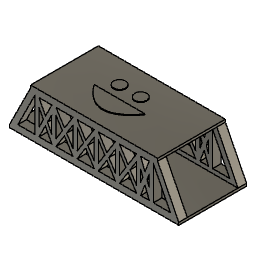
jason (Autodesk Fusion 360 design; units mm, degrees)
Autodesk Fusion 360 part; units mm, degrees
sketch "Sketch1" plane through (0, 0, 0) normal (0, 0, 1) x (1, 0, 0)
  line L0 (-100, 0) -> (-75, 50)
  line L1 (-75, 50) -> (75, 50)
  line L2 (75, 50) -> (100, 0)
  line L3 (100, 0) -> (-100, 0)
  line L4 (-70, 45) -> (-90, 5)
  line L5 (-90, 5) -> (90, 5)
  line L6 (90, 5) -> (70, 45)
  line L7 (70, 45) -> (-70, 45)
  line L8 (-70, 45) -> (-70, 5)
  line L9 (-50, 45) -> (-70, 5)
  line L10 (-50, 45) -> (-50, 5)
  line L11 (-50, 45) -> (-50, 5)
  line L12 (-50, 5) -> (-30, 45)
  line L13 (-30, 45) -> (-30, 5)
  line L14 (-10, 45) -> (-30, 5)
  line L15 (-10, 45) -> (-10, 5)
  line L16 (10, 45) -> (-10, 5)
  line L17 (10, 45) -> (10, 5)
  line L18 (10, 5) -> (30, 45)
  line L19 (30, 5) -> (30, 45)
  line L20 (30, 5) -> (50, 45)
  line L21 (50, 5) -> (50, 45)
  line L22 (70, 45) -> (50, 5)
  line L23 (70, 45) -> (70, 5)
  line L24 (-50, 5) -> (-60, 25)
  line L25 (-40, 25) -> (-30, 5)
  line L26 (-20, 25) -> (-10, 5)
  line L27 (0, 25) -> (10, 5)
  line L28 (20, 25) -> (30, 5)
  line L29 (40, 25) -> (50, 5)
  line L30 (60, 25) -> (70, 5)
  line L31 (80, 25) -> (70, 5)
  line L32 (-70, 6.8562) -> (-80, 25)
  line L33 (-70, 45) -> (-60, 25)
  line L34 (-50, 45) -> (-40, 25)
  line L35 (-30, 45) -> (-20, 25)
  line L36 (-10, 45) -> (0, 25)
  line L37 (10, 45) -> (20, 25)
  line L38 (30, 45) -> (40, 25)
  line L39 (50, 45) -> (60, 25)
  line L40 (-80, 25) -> (80, 25)
  constraint horizontal L1
  constraint parallel L1 L3
  constraint parallel L0 L4
  constraint parallel L3 L5
  constraint parallel L1 L7
  constraint coincident L5 L8.end
  constraint perpendicular L5 L8
  constraint coincident L7 L9.start
  constraint coincident L5 L10.end
  constraint perpendicular L5 L10
  constraint perpendicular L5 L11
  constraint coincident L7 L12.end
  constraint parallel L9 L12
  constraint coincident L5 L13.end
  constraint perpendicular L5 L13
  constraint coincident L7 L14.start
  constraint parallel L12 L14
  constraint coincident L5 L15.end
  constraint perpendicular L5 L15
  constraint coincident L7 L16.start
  constraint parallel L14 L16
  constraint coincident L5 L17.end
  constraint perpendicular L7 L17
  constraint coincident L7 L18.end
  constraint parallel L16 L18
  constraint coincident L5 L19.start
  constraint perpendicular L7 L19
  constraint coincident L7 L20.end
  constraint coincident L5 L21.start
  constraint perpendicular L7 L21
  constraint parallel L20 L22
  constraint coincident L5 L23.end
  constraint perpendicular L5 L23
  constraint midpoint L9 L24.end
  constraint midpoint L12 L25.start
  constraint midpoint L14 L26.start
  constraint midpoint L16 L27.start
  constraint midpoint L18 L28.start
  constraint midpoint L20 L29.start
  constraint parallel L28 L29
  constraint midpoint L22 L30.start
  constraint midpoint L6 L31.start
  constraint coincident L8 L32.start
  constraint midpoint L4 L32.end
extrude "Extrude1" add sketch "Sketch1" along normal blind 10 makes body 1
move_face "MoveFace1" to x (0.8, 0.4, -0.447214) y (0.4, 0.2, 0.894427) z (0.447214, -0.894427, 0) at (2.6343, -5.2686, 5.8905) 1 faces at (83.3333, 33.3333, 3.3333) on bodies 1
move_body "Move1" bodies 1 to x (1, 0, 0) y (0, 0, 1) z (0, -1, 0) at (0, 15, 5)
move_body "Move2" bodies 1 to x (1, 0, 0) y (0, 1, 0) z (0, 0, 1) at (0, -10, -5)
sketch "Sketch2" plane through (0, 0, 0) normal (0, 1, 0) x (1, 0, 0)
  line L0 (-70, -45) -> (-70, -5)
  line L1 (-70, -5) -> (-65, -5)
  line L2 (-65, -5) -> (-65, -45)
  line L3 (-65, -45) -> (-70, -45)
  line L4 (-65, -45) -> (-45, -5)
  line L5 (-45, -5) -> (-50, -5)
  line L6 (-50, -5) -> (-70, -45)
  line L7 (-45, -5) -> (-45, -45)
  line L8 (-45, -45) -> (-50, -45)
  line L9 (-50, -45) -> (-50, -5)
  line L10 (-70, -5) -> (-50, -45)
  line L11 (-45, -45) -> (-51.984, -45)
  line L12 (-65, -5) -> (-45, -45)
  line L13 (-70, -5) -> (-65, -5)
  line L14 (-45, -45) -> (-50, -45)
  line L15 (-50, -45) -> (-25, -5)
  line L16 (-25, -5) -> (-20, -5)
  line L17 (-20, -5) -> (-45, -45)
  line L18 (-25, -45) -> (-25, -5)
  line L19 (-20, -5) -> (-20, -45)
  line L20 (-20, -45) -> (-25, -45)
  line L21 (-25, -45) -> (-50, -5)
  line L22 (-20, -45) -> (-45, -5)
  line L23 (-25, -45) -> (0, -5)
  line L24 (0, -5) -> (5, -5)
  line L25 (5, -5) -> (-20, -45)
  line L26 (5, -5) -> (5, -45)
  line L27 (5, -45) -> (-20, -5)
  line L28 (-25, -5) -> (0, -45)
  line L29 (0, -45) -> (5, -45)
  line L30 (0, -5) -> (0, -45)
  line L31 (0, -45) -> (25, -5)
  line L32 (25, -5) -> (30, -5)
  line L33 (30, -5) -> (5, -45)
  line L34 (30, -5) -> (30, -45)
  line L35 (30, -45) -> (25, -45)
  line L36 (25, -45) -> (25, -5)
  line L37 (0, -5) -> (25, -45)
  line L38 (5, -5) -> (30, -45)
  line L39 (25, -45) -> (50, -5)
  line L40 (50, -5) -> (55, -5)
  line L41 (55, -5) -> (30, -45)
  line L42 (50, -45) -> (50, -5)
  line L43 (55, -5) -> (55, -45)
  line L44 (55, -45) -> (50, -45)
  line L45 (55, -45) -> (30, -5)
  line L46 (50, -45) -> (25, -5)
  line L47 (55, -5) -> (70, -45)
  line L48 (70, -45) -> (70, -5)
  line L49 (70, -5) -> (65, -5)
  line L50 (65, -5) -> (65, -45)
  line L51 (65, -45) -> (70, -45)
  line L52 (55, -45) -> (70, -5)
  line L53 (50, -45) -> (65, -5)
  line L54 (65, -45) -> (50, -5)
  constraint vertical L0
  constraint perpendicular L0 L1
  constraint perpendicular L1 L2
  constraint perpendicular L0 L3
  constraint perpendicular L0 L5
  constraint parallel L4 L6
  constraint perpendicular L5 L7
  constraint perpendicular L7 L8
  constraint perpendicular L5 L9
  constraint perpendicular L9 L11
  constraint perpendicular L9 L16
  constraint parallel L15 L17
  constraint perpendicular L16 L18
  constraint perpendicular L16 L19
  constraint perpendicular L18 L20
  constraint perpendicular L19 L24
  constraint parallel L23 L25
  constraint perpendicular L24 L26
  constraint parallel L27 L28
  constraint perpendicular L26 L29
  constraint perpendicular L30 L32
  constraint parallel L31 L33
  constraint perpendicular L32 L34
  constraint perpendicular L34 L35
  constraint perpendicular L32 L36
  constraint perpendicular L34 L40
  constraint parallel L39 L41
  constraint perpendicular L40 L42
  constraint perpendicular L40 L43
  constraint perpendicular L42 L44
  constraint parallel L43 L48
  constraint perpendicular L49 L50
  constraint perpendicular L43 L51
  constraint parallel L52 L53
extrude "Extrude2" add sketch "Sketch2" against normal blind 5 contours L2 L3 L6 | L0 L2 L6 L10 | L1 L2 L10 L13 | L2 L4 L6 L10 | L2 L6 L10 L12 | L4 L6 L10 L12 | L4 L9 L10 L12 | L4 L6 L9 L12 | L8 L11 L12 L14 L15 | L9 L12 L15 | L4 L9 L21 | L4 L5 L21 | L4 L7 L9 L12 L15 L21 | L7 L12 L15 | L7 L15 L17 L21 | L4 L7 L21 | L7 L15 L21 L22 | L15 L17 L21 L22 | L17 L18 L21 L22 | L15 L17 L18 L22 | L20 L22 L23 | L18 L22 L23 | L17 L18 L28 | L16 L17 L28 | L17 L18 L19 L22 L23 L28 | L19 L22 L23 | L19 L23 L25 L28 | L17 L19 L28 | L19 L23 L27 L28 | L23 L25 L27 L28 | L25 L27 L28 L30 | L23 L25 L27 L30 | L27 L29 L31 | L27 L30 L31 | L25 L30 L37 | L24 L25 L37 | L25 L26 L27 L30 L31 L37 | L26 L27 L31 | L26 L31 L33 L37 | L25 L26 L37 | L26 L31 L37 L38 | L31 L33 L37 L38 | L33 L36 L37 L38 | L31 L33 L36 L38 | L35 L38 L39 | L36 L38 L39 | L33 L36 L46 | L32 L33 L46 | L33 L34 L36 L38 L39 L46 | L34 L38 L39 | L34 L39 L41 L46 | L33 L34 L46 | L34 L39 L45 L46 | L39 L41 L45 L46 | L41 L42 L45 L46 | L39 L41 L42 L45 | L44 L45 L53 | L42 L45 L53 | L41 L42 L54 | L40 L41 L54 | L41 L42 L43 L45 L53 L54 | L43 L45 L53 | L43 L52 L53 L54 | L41 L43 L54 | L43 L47 L53 L54 | L47 L52 L53 L54 | L47 L50 L52 L54 | L47 L50 L52 L53 | L47 L50 L51 | L49 L50 L52 | L47 L48 L50 L52 bodies 1
extrude "Extrude3" add 1 faces at (68.3333, 0, 22.7778) along direction (0, 1, 0) blind 5 on bodies 1 bodies 1
copy_body "CopyPasteBodies2" bodies 1 makes body 2
move_body "Move4" bodies 2 to x (1, 0, 0) y (0, 1, 0) z (0, 0, 1) at (0, 60, 0)
sketch "Sketch3" plane through (0, 0, 0) normal (0, 0, 1) x (1, 0, 0)
move_body "Move5" bodies 2 to x (1, 0, 0) y (0, 1, 0) z (0, 0, 1) at (0, 10, 0)
sketch "Sketch4" plane through (0, 0, 0) normal (0, 0, 1) x (1, 0, 0)
  line L0 (-100, 70) -> (100, 70)
  line L1 (100, 70) -> (100, 0)
  line L2 (100, 0) -> (-100, 0)
  line L3 (-100, 0) -> (-100, 70)
  constraint horizontal L0
  constraint vertical L1
  constraint horizontal L2
  constraint vertical L3
extrude "Extrude4" add sketch "Sketch4" against normal blind 3 bodies 1 2
extrude "Extrude5" add 1 faces at (-33.3333, 70, -1) along direction (0, 1, 0) blind 5 on bodies 1 bodies 1
extrude "Extrude6" add 1 faces at (33.3333, 0, -1) along direction (0, -1, 0) blind 5 on bodies 1 bodies 1
sketch "Sketch5" plane through (0, 0, 0) normal (0, 0, 1) x (1, 0, 0)
  line L0 (80, -10, 50) -> (-80, -10, 50)
  line L1 (-80, -10, 50) -> (-80, 80, 50)
  line L2 (-80, 80, 50) -> (80, 80, 50)
  line L3 (80, 80, 50) -> (80, -10, 50)
sketch "Sketch6" plane through (0, 35, 50) normal (0, 0, 1) x (1, 0, 0)
extrude "Extrude7" add sketch "Sketch5" along normal blind 3 contours L0 L1 L2 L3 in plane through (0, 0, 50) normal (0, 0, 1) bodies 1
move_face "MoveFace2" by (0, -5, 0) 1 faces at (-26.6667, 80, 51) on bodies 1
move_face "MoveFace3" by (-5, 0, 0) 1 faces at (80, 46.6667, 51) on bodies 1
move_face "MoveFace4" by (0, 5, 0) 1 faces at (23.3333, -10, 52) on bodies 1
move_face "MoveFace5" by (5, 0, 0) 1 faces at (-80, 21.6667, 51) on bodies 1
sketch "Sketch7" plane through (0, 0, 0) normal (0, 0, 1) x (1, 0, 0)
  circle A0 centre (0, -40) radius 7.0711
  circle A1 centre (25, -40) radius 7.0711
  spline S0 degree 5 poles (-15, -55) (-14.4962, -55.7021) (-13.4782, -57.081) (-11.9195, -59.0734) (-9.778, -61.5771) (-6.9948, -64.4458) (-4.1055, -67.0409) (-1.1127, -69.3416) (1.9771, -71.3184) (5.1521, -72.9302) (8.3951, -74.1302) (11.6855, -74.8735) (15, -75.1261) (18.3145, -74.8735) (21.6049, -74.1302) (24.8479, -72.9302) (28.0229, -71.3184) (31.1127, -69.3416) (34.1055, -67.0409) (36.9948, -64.4458) (39.778, -61.5771) (41.9195, -59.0734) (43.4782, -57.081) (44.4962, -55.7021) (45, -55) knots 0 0 0 0 0 0 0.05 0.1 0.15 0.2 0.25 0.3 0.35 0.4 0.45 0.5 0.55 0.6 0.65 0.7 0.75 0.8 0.85 0.9 0.95 1 1 1 1 1 1
  line L0 (-15, -55) -> (45, -55)
  point P0 (0, -70)
  point P1 (15, -75)
  point P2 (30, -70)
  constraint horizontal L0
extrude "Extrude8" add sketch "Sketch7" along normal blind 1 separate body makes body 3 at (26.8062, -41.9466, 0) makes body 4 at (-3.9871, -41.4806, 0) makes body 5 at (5.9471, -58.9238, 0)
move_body "Move6" bodies 5 3 4 to x (1, 0, 0) y (0, 1, 0) z (0, 0, 1) at (-20, 85, 55)
